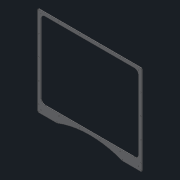
# Autodesk Inventor part: left_plate_01
Saved by Autodesk Inventor 2022 (Build 260153000, 153)
## iProperties
Created: 2025-01-09
Part Number: left_plate_01
Material: 一般
Document SubType Name: Modeling
Designer: nyxeon
Density: 1 g/cm^3
Appearance: 既定
Author: nyxeon
Autodesk Inventor part; units mm, degrees
ref_plane "YZ Plane" through (0, 0, 0) normal (1, 0, 0) x (0, 1, 0)
ref_plane "XZ Plane" through (0, 0, 0) normal (0, 1, 0) x (-1, 0, 0)
ref_plane "XY Plane" through (0, 0, 0) normal (0, 0, 1) x (1, 0, 0)
sketch "スケッチ1" plane through (0, 0, 0) normal (0, 0, 1) x (1, 0, 0)
  circle A0 centre (-490.19, 90.19) radius 2.1 projected
  circle A1 centre (-490.19, 290.19) radius 2.1 projected
  circle A2 centre (-190.19, 390.19) radius 2.1 projected
  circle A3 centre (-390.19, 390.19) radius 2.1 projected
  circle A4 centre (-290.19, -9.81) radius 2.1 projected
  circle A5 centre (-90.19, -9.81) radius 2.1 projected
  circle A6 centre (9.81, 190.19) radius 2.1 projected
  circle A7 centre (9.81, 390.19) radius 2.1 projected
  circle A8 centre (-490.19, -9.81) radius 2.1 projected
  circle A9 centre (-233.68, 12.7) radius 1.6 construction
  circle A10 centre (-29.21, 294.64) radius 1.6 construction
  circle A11 centre (-161.29, 294.64) radius 1.6 construction
  circle A12 centre (-233.68, 294.64) radius 1.6 construction
  circle A13 centre (-233.68, 137.16) radius 1.6 construction
  circle A14 centre (-161.29, 137.16) radius 1.6 construction
  circle A15 centre (-6.35, 137.16) radius 1.6 construction
  circle A16 centre (-6.35, 12.7) radius 1.6 construction
  circle A17 centre (-161.29, 12.7) radius 1.6 construction
  circle A18 centre (9.81, -9.81) radius 2.1 projected
  circle A19 centre (-490.19, 390.19) radius 2.1 projected
  circle A20 centre (9.81, 290.19) radius 2.1 projected
  circle A21 centre (9.81, 90.19) radius 2.1
  circle A22 centre (-190.19, -9.81) radius 2.1 projected
  circle A23 centre (-390.19, -9.81) radius 2.1 projected
  circle A24 centre (-290.19, 390.19) radius 2.1 projected
  circle A25 centre (-90.19, 390.19) radius 2.1 projected
  circle A26 centre (-490.19, 190.19) radius 2.1 projected
  line L0 (-21.19, 1.19) -> (-459.19, 1.19)
  line L1 (-479.19, 21.19) -> (-479.19, 359.19)
  line L2 (-459.19, 379.19) -> (-21.19, 379.19)
  line L3 (-1.19, 359.19) -> (-1.19, 21.19)
  circle A27 centre (9.81, -9.81) radius 5
  circle A28 centre (9.81, -9.81) radius 15.5563 construction
  line L4 (9.81, -9.81) -> (-1.19, 1.19) construction
  line L5 (9.81, -9.81) -> (25.3663, -9.81) construction
  circle A29 centre (-1.19, 1.19) radius 5 construction
  circle A30 centre (-1.19, 1.19) radius 2.1
  line L6 (-240.19, 1.19) -> (-240.19, 379.19) construction
  line L7 (-1.19, 190.19) -> (-479.19, 190.19) construction
  circle A31 centre (-1.19, 379.19) radius 2.1
  circle A32 centre (-479.19, 1.19) radius 2.1
  circle A33 centre (-479.19, 379.19) radius 2.1
  arc A34 (-1.19, 359.19) -> (-21.19, 379.19) centre (-21.19, 359.19) ccw
  arc A35 (-459.19, 379.19) -> (-479.19, 359.19) centre (-459.19, 359.19) ccw
  arc A36 (-479.19, 21.19) -> (-459.19, 1.19) centre (-459.19, 21.19) ccw
  arc A37 (-21.19, 1.19) -> (-1.19, 21.19) centre (-21.19, 21.19) ccw
  line L8 (9.81, -4.81) -> (-11.2166, -4.81) construction
  arc A38 (-483.7257, 425.19) -> (-483.7257, -44.81) centre (161.4767, 190.19) ccw projected
  line L9 (-483.7257, 425.19) -> (-379.99, 425.19) projected
  arc A39 (-379.99, 425.19) -> (-100.39, 425.19) centre (-240.19, 735.924) ccw projected
  line L10 (-100.39, 425.19) -> (3.3457, 425.19) projected
  arc A40 (3.3457, -44.81) -> (3.3457, 425.19) centre (-641.8567, 190.19) ccw projected
  line L11 (3.3457, -44.81) -> (-79.99, -44.81) projected
  arc A41 (-79.99, -44.81) -> (-400.39, -44.81) centre (-240.19, -457.544) ccw projected
  line L12 (-400.39, -44.81) -> (-483.7257, -44.81) projected
  arc A42 (14.81, 390.19) -> (9.81, 395.19) centre (9.81, 390.19) ccw
  line L13 (9.81, 395.19) -> (-490.19, 395.19)
  line L14 (14.81, -9.81) -> (14.81, 390.19)
  arc A43 (9.81, -14.81) -> (14.81, -9.81) centre (9.81, -9.81) ccw construction
  line L15 (-490.19, -14.81) -> (9.81, -14.81)
  arc A44 (-495.19, -9.81) -> (-490.19, -14.81) centre (-490.19, -9.81) ccw
  line L16 (-495.19, 390.19) -> (-495.19, -9.81)
  arc A45 (-490.19, 395.19) -> (-495.19, 390.19) centre (-490.19, 390.19) ccw
  point P0 (0, 0)
  point P1 (-1.19, 1.19)
  point P2 (-479.19, 379.19)
  point P3 (-479.19, 1.19)
  point P4 (-1.19, 379.19)
  point P5 (14.59, -11.277)
  point P6 (-494.97, 391.657)
  point P7 (-494.97, -11.277)
  dimension "d4" = 31.1127
  dimension "d5" = 135
  dimension "d6" = 10
  dimension "d10" = 20
  dimension "d11" = 6
  dimension "d14" = 11
  dimension "d15" = 11
  dimension "d16" = 11
  dimension "d17" = 11
  dimension "d18" = 11
  dimension "d30" = 100
  constraints: 26 end point, 17 point on circle, 15 centre point, 9 tangent, 8 point on line, 5 equal radius, 5 horizontal, 4 coincident, 4 midpoint, 3 symmetric about line, 2 parallel, 2 vertical, 1 equal length, 1 perpendicular, 1 vertical alignment, 22 other
  measures "d5" angle of L5 L4
  measures "d6" diameter of A29
  measures "d10" radius of A34
  measures "d11" distance from line of L8 L4.end
  measures "d14" distance from line of A7.centre L2
  measures "d15" distance from line of A7.centre L3
  measures "d16" distance from line of L0 A18.centre
  measures "d17" horizontal distance of A18.centre A30.centre
  measures "d18" distance from line of A8.centre L1
  measures "d30" distance of A21.centre A6.centre
extrude "押し出し1" add sketch "スケッチ1" against normal blind 3 contours A27 | A27 L15 A44 L16 A45 L13 A42 L14 | A27 A40 L11 A41 L15 | A41 L12 A38 A44 L15 | A30 | A32
sketch "スケッチ3" plane through (0, 0, -3) normal (0, 0, -1) x (-1, 0, 0)
  arc A0 (-14.81, -9.81) -> (-14.59, -11.277) centre (-9.81, -9.81) ccw projected
  arc A1 (-14.59, -11.277) -> (-3.3457, -44.81) centre (641.8567, 190.19) ccw projected
  arc A2 (483.7257, -44.81) -> (494.97, -11.277) centre (-161.4767, 190.19) ccw projected
  arc A3 (494.97, -11.277) -> (495.19, -9.81) centre (490.19, -9.81) ccw projected
  line L0 (-14.81, -9.81) -> (-14.81, -39.81)
  arc A4 (-14.81, -39.81) -> (-9.81, -44.81) centre (-9.81, -39.81) ccw
  line L1 (79.99, -44.81) -> (-3.3457, -44.81) projected
  line L2 (-9.81, -44.81) -> (-3.3457, -44.81)
  line L3 (495.19, -9.81) -> (495.19, -39.81)
  arc A5 (490.19, -44.81) -> (495.19, -39.81) centre (490.19, -39.81) ccw
  line L4 (490.19, -44.81) -> (483.7257, -44.81)
  point P0 (0, 0)
  dimension "d19" = 5
  constraints: 8 end point, 4 point on circle, 4 tangent, 2 centre point, 2 perpendicular, 2 vertical, 1 equal radius
  measures "d19" radius of A4
extrude "押し出し3" add sketch "スケッチ3" against normal up to surface (3 mm away)
fillet "フィレット2" radius 5 2 edges at (-79.99, -44.81, -1.5) (-400.39, -44.81, -1.5)
sketch "スケッチ4" plane through (0, 0, -3) normal (0, 0, -1) x (-1, 0, 0)
  arc A0 (-14.81, -39.81) -> (-9.81, -44.81) centre (-9.81, -39.81) ccw construction
  circle A1 centre (-9.81, -9.81) radius 2.1 construction
  arc A2 (490.19, -44.81) -> (495.19, -39.81) centre (490.19, -39.81) ccw construction
  circle A3 centre (490.19, -9.81) radius 2.1 construction
  line L0 (-9.81, -9.81) -> (1.19, 1.19) construction
  line L1 (1.19, 1.19) -> (1.19, -28.81) construction
  line L2 (1.19, -28.81) -> (-9.81, -39.81) construction
  line L3 (-9.81, -39.81) -> (-9.81, -9.81) construction
  line L4 (479.19, 1.19) -> (490.19, -9.81) construction
  line L5 (490.19, -9.81) -> (490.19, -39.81) construction
  line L6 (490.19, -39.81) -> (479.19, -28.81) construction
  line L7 (479.19, -28.81) -> (479.19, 1.19) construction
  circle A4 centre (-9.81, -39.81) radius 2.1
  circle A5 centre (490.19, -39.81) radius 2.1
  arc A6 (79.0564, -44.81) -> (80.8558, -44.475) centre (79.0564, -39.81) ccw construction
  arc A7 (399.5242, -44.475) -> (401.3236, -44.81) centre (401.3236, -39.81) ccw construction
  circle A8 centre (401.3236, -39.81) radius 2.1
  circle A9 centre (79.0564, -39.81) radius 2.1
  circle A10 centre (1.19, -28.81) radius 2.1
  circle A11 centre (479.19, -28.81) radius 2.1
  dimension "d27" = 11
  dimension "d28" = 11
  dimension "d29" = 45
  constraints: 16 end point, 6 centre point, 6 coincident, 6 equal radius, 5 parallel, 1 perpendicular, 1 vertical
  measures "d27" distance from line of L4.end L7
  measures "d28" horizontal distance of L0.end L0.start
  measures "d29" angle of L2 L3
extrude "押し出し4" cut sketch "スケッチ4" against normal through all
